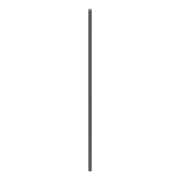
# Autodesk Inventor part: Part5
Saved by Autodesk Inventor 2016 (Build 200138000, 138)
## iProperties
Created: 2016-03-29
Part Number: Part5
Material: Stainless Steel
Document SubType Name: Modeling
Designer: admin
Density: 1 g/cm^3
Appearance: Semi-Polished
Author: admin
Autodesk Inventor part; units mm, degrees
ref_plane "YZ Plane" through (0, 0, 0) normal (1, 0, 0) x (0, 1, 0)
ref_plane "XZ Plane" through (0, 0, 0) normal (0, 1, 0) x (-1, 0, 0)
ref_plane "XY Plane" through (0, 0, 0) normal (0, 0, 1) x (1, 0, 0)
sketch "Sketch1" plane through (0, 0, 0) normal (0, 0, 1) x (1, 0, 0)
  circle A0 centre (-28, -169.4449) radius 2 projected
  circle A1 centre (-28, -169.4449) radius 5
  point P0 (0, 0)
  dimension "d0" = 10
  constraints: 1 centre point, 1 coincident
  measures "d0" diameter of A1
extrude "Extrusion1" add sketch "Sketch1" along normal blind 533 contours A0 | A1
sketch "Sketch2" plane through (-28, -169.4449, 533) normal (0, 0, 1) x (1, 0, 0)
  circle A0 centre (0, 0) radius 5 projected
  point P0 (28, 169.4449)
hole "Hole1" at (-28, -169.4449, 533) direction (0, 0, -1) diameter 3.242 depth 17 tip angle 118 thread size "M4x0.7" class "6H" standard "ISO Metric profile"
sketch "Sketch3" plane through (-28, -169.4449, 0) normal (0, 0, -1) x (-1, 0, 0)
  circle A0 centre (0, 0) radius 5 projected
  point P0 (-28, 169.4449)
hole "Hole2" at (-28, -169.4449, 0) direction (0, 0, 1) diameter 3.242 depth 17 tip angle 118 thread size "M4x0.7" class "6H" standard "ISO Metric profile"
chamfer "Chamfer1" distance 0.2 angle 45 2 edges at (-33, -169.4449, 0) (-33, -169.4449, 533)
body "Solid1"
